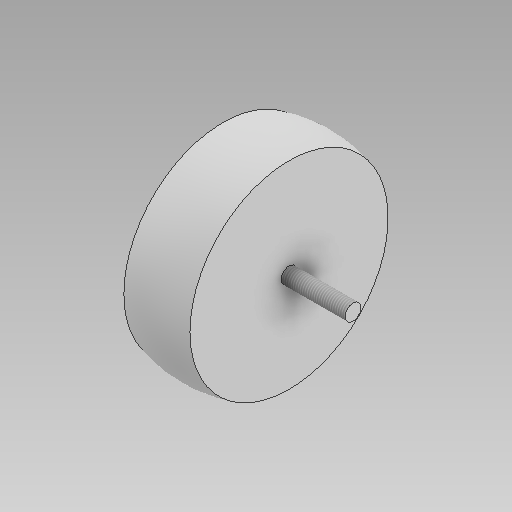
# Autodesk Inventor part: 6inch_wheel
Saved by Autodesk Inventor 2021.2 (Build 252289000, 289)
## iProperties
Created: 2021-05-27
Part Number: 6inch_wheel
Material: Generic
Document SubType Name: Modeling
Designer: gisen
Density: 1 g/cm^3
Appearance: Default
Author: gisen
Autodesk Inventor part; units mm, degrees
ref_plane "YZ Plane" through (0, 0, 0) normal (1, 0, 0) x (0, 1, 0)
ref_plane "XZ Plane" through (0, 0, 0) normal (0, 1, 0) x (-1, 0, 0)
ref_plane "XY Plane" through (0, 0, 0) normal (0, 0, 1) x (1, 0, 0)
sketch "スケッチ2" plane through (0, 0, 0) normal (0, 1, 0) x (-1, 0, 0)
  line L0 (-25, 0) -> (25, 0)
  line L1 (25, 0) -> (25, 75)
  line L2 (25, 75) -> (-25, 75)
  line L3 (-25, 75) -> (-25, 0)
  line L4 (0, -30.7429) -> (0, 96.7071) construction
  arc A0 (25, 75) -> (-25, 75) centre (0, -12.5357) ccw
  line L5 (35, 0) -> (-35, 0) construction
  point P0 (0, 0)
  dimension "d0" = 78.5
  dimension "d1" = 75
  dimension "d2" = 50
  constraints: 8 end point, 2 parallel, 2 point on circle, 1 centre point, 1 collinear, 1 horizontal, 1 perpendicular, 1 other
  measures "d0" distance edge to line of A0 L0
  measures "d1" distance between parallel lines of L0 L2
  measures "d2" distance between parallel lines of L1 L3
revolve "回転1" add sketch "スケッチ2" angle 360 about axis through (-10, 0, 0) along (1, 0, 0)
sketch "スケッチ3" plane through (0, 0, 0) normal (1, 0, 0) x (0, 1, 0)
  point P0 (0, 0)
sketch "スケッチ4" plane through (0, 0, 0) normal (1, 0, 0) x (0, 1, 0)
  circle A0 centre (0, 0) radius 6
  dimension "d4" = 12
  constraints: 1 centre point, 1 coincident
  measures "d4" diameter of A0
extrude "押し出し1" add sketch "スケッチ4" along normal mid plane 147
thread "ねじ1" size "M12x1.75" class "6g" standard "ANSI Metric M Profile" full length
equation "\"d0\" = 0.5 * D"
equation "\"D\" = 157"
